Autodesk Fusion 360 part; units mm, degrees
(part 4 of 7)
  spline S11 degree 5 poles (-8.4802, -4.8873) (-8.4781, -4.8839) (-8.474, -4.8771) (-8.4679, -4.8668) (-8.4597, -4.8532) (-8.4496, -4.8361) (-8.4397, -4.8189) (-8.4298, -4.8018) (-8.42, -4.7846) (-8.4104, -4.7674) (-8.4008, -4.7502) (-8.3914, -4.733) (-8.3821, -4.7158) (-8.3729, -4.6985) (-8.3638, -4.6813) (-8.3548, -4.664) (-8.3459, -4.6467) (-8.3371, -4.6293) (-8.3285, -4.612) (-8.3199, -4.5947) (-8.3115, -4.5773) (-8.3032, -4.5599) (-8.295, -4.5426) (-8.2869, -4.5252) (-8.279, -4.5077) (-8.2711, -4.4903) (-8.2634, -4.4729) (-8.2558, -4.4554) (-8.2483, -4.438) (-8.241, -4.4205) (-8.2337, -4.403) (-8.2266, -4.3856) (-8.2196, -4.3681) (-8.2128, -4.3506) (-8.2061, -4.3331) (-8.1995, -4.3155) (-8.193, -4.298) (-8.1866, -4.2805) (-8.1804, -4.2629) (-8.1743, -4.2454) (-8.1684, -4.2279) (-8.1626, -4.2103) (-8.1569, -4.1928) (-8.1514, -4.1752) (-8.146, -4.1576) (-8.1408, -4.1401) (-8.1357, -4.1225) (-8.1307, -4.1049) (-8.1259, -4.0874) (-8.1212, -4.0698) (-8.1167, -4.0522) (-8.1124, -4.0347) (-8.1082, -4.0171) (-8.1042, -3.9995) (-8.1004, -3.982) (-8.0967, -3.9644) (-8.0932, -3.9469) (-8.0898, -3.9293) (-8.0866, -3.9118) (-8.0836, -3.8943) (-8.0808, -3.8768) (-8.0783, -3.8592) (-8.076, -3.8417) (-8.074, -3.8243) (-8.0722, -3.8068) (-8.0706, -3.7893) (-8.0691, -3.7719) (-8.0678, -3.7545) (-8.0667, -3.7371) (-8.0658, -3.7197) (-8.0656, -3.7024) (-8.066, -3.6885) (-8.0667, -3.6782) (-8.0674, -3.6713) (-8.0678, -3.6679) knots -1 -1 -1 -1 -1 -1 -0.98571429 -0.97142857 -0.95714286 -0.94285714 -0.92857143 -0.91428571 -0.9 -0.88571429 -0.87142857 -0.85714286 -0.84285714 -0.82857143 -0.81428571 -0.8 -0.78571429 -0.77142857 -0.75714286 -0.74285714 -0.72857143 -0.71428571 -0.7 -0.68571429 -0.67142857 -0.65714286 -0.64285714 -0.62857143 -0.61428571 -0.6 -0.58571429 -0.57142857 -0.55714286 -0.54285714 -0.52857143 -0.51428571 -0.5 -0.48571429 -0.47142857 -0.45714286 -0.44285714 -0.42857143 -0.41428571 -0.4 -0.38571429 -0.37142857 -0.35714286 -0.34285714 -0.32857143 -0.31428571 -0.3 -0.28571429 -0.27142857 -0.25714286 -0.24285714 -0.22857143 -0.21428571 -0.2 -0.18571429 -0.17142857 -0.15714286 -0.14285714 -0.12857143 -0.11428571 -0.1 -0.08571429 -0.07142857 -0.05714286 -0.04285714 -0.02857143 -0.01428571 0 0 0 0 0 0
  line L17 (-8.0678, -3.6679) -> (-8.1065, -3.3269)
  arc A18 (-7.9374, -3.1065) -> (-8.1065, -3.3269) centre (-7.9078, -3.3043) ccw
  line L18 (-7.9374, -3.1065) -> (-7.0422, -3.1065)
  arc A19 (-6.8731, -3.3269) -> (-7.0422, -3.1065) centre (-7.0718, -3.3043) ccw
  line L19 (-6.8731, -3.3269) -> (-6.9118, -3.6679)
  spline S12 degree 5 poles (-6.9118, -3.6679) (-6.9122, -3.6713) (-6.9128, -3.6782) (-6.9136, -3.6885) (-6.914, -3.7024) (-6.9138, -3.7197) (-6.9129, -3.7371) (-6.9118, -3.7545) (-6.9105, -3.7719) (-6.909, -3.7893) (-6.9074, -3.8068) (-6.9056, -3.8243) (-6.9036, -3.8417) (-6.9013, -3.8592) (-6.8988, -3.8768) (-6.896, -3.8943) (-6.893, -3.9118) (-6.8898, -3.9293) (-6.8864, -3.9469) (-6.8829, -3.9644) (-6.8792, -3.982) (-6.8754, -3.9995) (-6.8714, -4.0171) (-6.8672, -4.0347) (-6.8629, -4.0522) (-6.8584, -4.0698) (-6.8537, -4.0874) (-6.8489, -4.1049) (-6.8439, -4.1225) (-6.8388, -4.1401) (-6.8336, -4.1576) (-6.8282, -4.1752) (-6.8227, -4.1928) (-6.817, -4.2103) (-6.8112, -4.2279) (-6.8053, -4.2454) (-6.7992, -4.2629) (-6.793, -4.2805) (-6.7866, -4.298) (-6.7801, -4.3155) (-6.7735, -4.3331) (-6.7668, -4.3506) (-6.76, -4.3681) (-6.753, -4.3856) (-6.7459, -4.403) (-6.7386, -4.4205) (-6.7313, -4.438) (-6.7238, -4.4554) (-6.7162, -4.4729) (-6.7085, -4.4903) (-6.7006, -4.5077) (-6.6927, -4.5252) (-6.6846, -4.5426) (-6.6764, -4.5599) (-6.6681, -4.5773) (-6.6597, -4.5947) (-6.6511, -4.612) (-6.6425, -4.6293) (-6.6337, -4.6467) (-6.6248, -4.664) (-6.6158, -4.6813) (-6.6067, -4.6985) (-6.5975, -4.7158) (-6.5882, -4.733) (-6.5788, -4.7502) (-6.5692, -4.7674) (-6.5596, -4.7846) (-6.5498, -4.8018) (-6.5399, -4.8189) (-6.53, -4.8361) (-6.5199, -4.8532) (-6.5117, -4.8668) (-6.5056, -4.8771) (-6.5015, -4.8839) (-6.4994, -4.8873) knots 0 0 0 0 0 0 0.01428571 0.02857143 0.04285714 0.05714286 0.07142857 0.08571429 0.1 0.11428571 0.12857143 0.14285714 0.15714286 0.17142857 0.18571429 0.2 0.21428571 0.22857143 0.24285714 0.25714286 0.27142857 0.28571429 0.3 0.31428571 0.32857143 0.34285714 0.35714286 0.37142857 0.38571429 0.4 0.41428571 0.42857143 0.44285714 0.45714286 0.47142857 0.48571429 0.5 0.51428571 0.52857143 0.54285714 0.55714286 0.57142857 0.58571429 0.6 0.61428571 0.62857143 0.64285714 0.65714286 0.67142857 0.68571429 0.7 0.71428571 0.72857143 0.74285714 0.75714286 0.77142857 0.78571429 0.8 0.81428571 0.82857143 0.84285714 0.85714286 0.87142857 0.88571429 0.9 0.91428571 0.92857143 0.94285714 0.95714286 0.97142857 0.98571429 1 1 1 1 1 1
  arc A20 (-6.4994, -4.8873) -> (-5.9669, -4.8873) centre (-6.2332, 2.3078) ccw
  spline S13 degree 5 poles (-5.9669, -4.8873) (-5.9649, -4.8839) (-5.9607, -4.8771) (-5.9546, -4.8668) (-5.9464, -4.8532) (-5.9364, -4.8361) (-5.9264, -4.8189) (-5.9165, -4.8018) (-5.9067, -4.7846) (-5.8971, -4.7674) (-5.8876, -4.7502) (-5.8781, -4.733) (-5.8688, -4.7158) (-5.8596, -4.6985) (-5.8505, -4.6813) (-5.8415, -4.664) (-5.8326, -4.6467) (-5.8238, -4.6293) (-5.8152, -4.612) (-5.8067, -4.5947) (-5.7982, -4.5773) (-5.7899, -4.5599) (-5.7817, -4.5426) (-5.7737, -4.5252) (-5.7657, -4.5077) (-5.7579, -4.4903) (-5.7501, -4.4729) (-5.7425, -4.4554) (-5.7351, -4.438) (-5.7277, -4.4205) (-5.7205, -4.403) (-5.7134, -4.3856) (-5.7064, -4.3681) (-5.6995, -4.3506) (-5.6928, -4.3331) (-5.6862, -4.3155) (-5.6797, -4.298) (-5.6734, -4.2805) (-5.6672, -4.2629) (-5.6611, -4.2454) (-5.6551, -4.2279) (-5.6493, -4.2103) (-5.6437, -4.1928) (-5.6381, -4.1752) (-5.6327, -4.1576) (-5.6275, -4.1401) (-5.6224, -4.1225) (-5.6174, -4.1049) (-5.6126, -4.0874) (-5.608, -4.0698) (-5.6035, -4.0522) (-5.5991, -4.0347) (-5.5949, -4.0171) (-5.5909, -3.9995) (-5.5871, -3.982) (-5.5835, -3.9644) (-5.5799, -3.9469) (-5.5766, -3.9293) (-5.5734, -3.9118) (-5.5703, -3.8943) (-5.5675, -3.8768) (-5.565, -3.8592) (-5.5627, -3.8417) (-5.5607, -3.8243) (-5.5589, -3.8068) (-5.5573, -3.7893) (-5.5559, -3.7719) (-5.5545, -3.7545) (-5.5534, -3.7371) (-5.5526, -3.7197) (-5.5523, -3.7024) (-5.5527, -3.6885) (-5.5535, -3.6782) (-5.5542, -3.6713) (-5.5545, -3.6679) knots -1 -1 -1 -1 -1 -1 -0.98571429 -0.97142857 -0.95714286 -0.94285714 -0.92857143 -0.91428571 -0.9 -0.88571429 -0.87142857 -0.85714286 -0.84285714 -0.82857143 -0.81428571 -0.8 -0.78571429 -0.77142857 -0.75714286 -0.74285714 -0.72857143 -0.71428571 -0.7 -0.68571429 -0.67142857 -0.65714286 -0.64285714 -0.62857143 -0.61428571 -0.6 -0.58571429 -0.57142857 -0.55714286 -0.54285714 -0.52857143 -0.51428571 -0.5 -0.48571429 -0.47142857 -0.45714286 -0.44285714 -0.42857143 -0.41428571 -0.4 -0.38571429 -0.37142857 -0.35714286 -0.34285714 -0.32857143 -0.31428571 -0.3 -0.28571429 -0.27142857 -0.25714286 -0.24285714 -0.22857143 -0.21428571 -0.2 -0.18571429 -0.17142857 -0.15714286 -0.14285714 -0.12857143 -0.11428571 -0.1 -0.08571429 -0.07142857 -0.05714286 -0.04285714 -0.02857143 -0.01428571 0 0 0 0 0 0
  line L20 (-5.5545, -3.6679) -> (-5.5933, -3.3269)
  arc A21 (-5.4241, -3.1065) -> (-5.5933, -3.3269) centre (-5.3945, -3.3043) ccw
  line L21 (-5.4241, -3.1065) -> (-4.5289, -3.1065)
  arc A22 (-4.3598, -3.3269) -> (-4.5289, -3.1065) centre (-4.5585, -3.3043) ccw
  line L22 (-4.3598, -3.3269) -> (-4.3985, -3.6679)
  spline S14 degree 5 poles (-4.3985, -3.6679) (-4.3989, -3.6713) (-4.3996, -3.6782) (-4.4003, -3.6885) (-4.4007, -3.7024) (-4.4005, -3.7197) (-4.3997, -3.7371) (-4.3985, -3.7545) (-4.3972, -3.7719) (-4.3957, -3.7893) (-4.3941, -3.8068) (-4.3923, -3.8243) (-4.3903, -3.8417) (-4.3881, -3.8592) (-4.3855, -3.8768) (-4.3827, -3.8943) (-4.3797, -3.9118) (-4.3765, -3.9293) (-4.3731, -3.9469) (-4.3696, -3.9644) (-4.3659, -3.982) (-4.3621, -3.9995) (-4.3581, -4.0171) (-4.3539, -4.0347) (-4.3496, -4.0522) (-4.3451, -4.0698) (-4.3404, -4.0874) (-4.3356, -4.1049) (-4.3307, -4.1225) (-4.3255, -4.1401) (-4.3203, -4.1576) (-4.3149, -4.1752) (-4.3094, -4.1928) (-4.3037, -4.2103) (-4.2979, -4.2279) (-4.292, -4.2454) (-4.2859, -4.2629) (-4.2797, -4.2805) (-4.2733, -4.298) (-4.2669, -4.3155) (-4.2603, -4.3331) (-4.2535, -4.3506) (-4.2467, -4.3681) (-4.2397, -4.3856) (-4.2326, -4.403) (-4.2253, -4.4205) (-4.218, -4.438) (-4.2105, -4.4554) (-4.2029, -4.4729) (-4.1952, -4.4903) (-4.1874, -4.5077) (-4.1794, -4.5252) (-4.1713, -4.5426) (-4.1631, -4.5599) (-4.1548, -4.5773) (-4.1464, -4.5947) (-4.1379, -4.612) (-4.1292, -4.6293) (-4.1204, -4.6467) (-4.1116, -4.664) (-4.1026, -4.6813) (-4.0935, -4.6985) (-4.0843, -4.7158) (-4.0749, -4.733) (-4.0655, -4.7502) (-4.056, -4.7674) (-4.0463, -4.7846) (-4.0365, -4.8018) (-4.0267, -4.8189) (-4.0167, -4.8361) (-4.0066, -4.8532) (-3.9985, -4.8668) (-3.9923, -4.8771) (-3.9882, -4.8839) (-3.9861, -4.8873) knots 0 0 0 0 0 0 0.01428571 0.02857143 0.04285714 0.05714286 0.07142857 0.08571429 0.1 0.11428571 0.12857143 0.14285714 0.15714286 0.17142857 0.18571429 0.2 0.21428571 0.22857143 0.24285714 0.25714286 0.27142857 0.28571429 0.3 0.31428571 0.32857143 0.34285714 0.35714286 0.37142857 0.38571429 0.4 0.41428571 0.42857143 0.44285714 0.45714286 0.47142857 0.48571429 0.5 0.51428571 0.52857143 0.54285714 0.55714286 0.57142857 0.58571429 0.6 0.61428571 0.62857143 0.64285714 0.65714286 0.67142857 0.68571429 0.7 0.71428571 0.72857143 0.74285714 0.75714286 0.77142857 0.78571429 0.8 0.81428571 0.82857143 0.84285714 0.85714286 0.87142857 0.88571429 0.9 0.91428571 0.92857143 0.94285714 0.95714286 0.97142857 0.98571429 1 1 1 1 1 1
  arc A23 (-3.9861, -4.8873) -> (-3.4537, -4.8873) centre (-3.7199, 2.3078) ccw
  spline S15 degree 5 poles (-3.4537, -4.8873) (-3.4516, -4.8839) (-3.4475, -4.8771) (-3.4413, -4.8668) (-3.4332, -4.8532) (-3.4231, -4.8361) (-3.4131, -4.8189) (-3.4032, -4.8018) (-3.3935, -4.7846) (-3.3838, -4.7674) (-3.3743, -4.7502) (-3.3648, -4.733) (-3.3555, -4.7158) (-3.3463, -4.6985) (-3.3372, -4.6813) (-3.3282, -4.664) (-3.3193, -4.6467) (-3.3106, -4.6293) (-3.3019, -4.612) (-3.2934, -4.5947) (-3.285, -4.5773) (-3.2766, -4.5599) (-3.2685, -4.5426) (-3.2604, -4.5252) (-3.2524, -4.5077) (-3.2446, -4.4903) (-3.2369, -4.4729) (-3.2293, -4.4554) (-3.2218, -4.438) (-3.2144, -4.4205) (-3.2072, -4.403) (-3.2001, -4.3856) (-3.1931, -4.3681) (-3.1862, -4.3506) (-3.1795, -4.3331) (-3.1729, -4.3155) (-3.1664, -4.298) (-3.1601, -4.2805) (-3.1539, -4.2629) (-3.1478, -4.2454) (-3.1419, -4.2279) (-3.136, -4.2103) (-3.1304, -4.1928) (-3.1249, -4.1752) (-3.1195, -4.1576) (-3.1142, -4.1401) (-3.1091, -4.1225) (-3.1042, -4.1049) (-3.0993, -4.0874) (-3.0947, -4.0698) (-3.0902, -4.0522) (-3.0858, -4.0347) (-3.0817, -4.0171) (-3.0777, -3.9995) (-3.0738, -3.982) (-3.0702, -3.9644) (-3.0667, -3.9469) (-3.0633, -3.9293) (-3.0601, -3.9118) (-3.0571, -3.8943) (-3.0543, -3.8768) (-3.0517, -3.8592) (-3.0495, -3.8417) (-3.0474, -3.8243) (-3.0457, -3.8068) (-3.0441, -3.7893) (-3.0426, -3.7719) (-3.0413, -3.7545) (-3.0401, -3.7371) (-3.0393, -3.7197) (-3.0391, -3.7024) (-3.0395, -3.6885) (-3.0402, -3.6782) (-3.0409, -3.6713) (-3.0413, -3.6679) knots -1 -1 -1 -1 -1 -1 -0.98571429 -0.97142857 -0.95714286 -0.94285714 -0.92857143 -0.91428571 -0.9 -0.88571429 -0.87142857 -0.85714286 -0.84285714 -0.82857143 -0.81428571 -0.8 -0.78571429 -0.77142857 -0.75714286 -0.74285714 -0.72857143 -0.71428571 -0.7 -0.68571429 -0.67142857 -0.65714286 -0.64285714 -0.62857143 -0.61428571 -0.6 -0.58571429 -0.57142857 -0.55714286 -0.54285714 -0.52857143 -0.51428571 -0.5 -0.48571429 -0.47142857 -0.45714286 -0.44285714 -0.42857143 -0.41428571 -0.4 -0.38571429 -0.37142857 -0.35714286 -0.34285714 -0.32857143 -0.31428571 -0.3 -0.28571429 -0.27142857 -0.25714286 -0.24285714 -0.22857143 -0.21428571 -0.2 -0.18571429 -0.17142857 -0.15714286 -0.14285714 -0.12857143 -0.11428571 -0.1 -0.08571429 -0.07142857 -0.05714286 -0.04285714 -0.02857143 -0.01428571 0 0 0 0 0 0
  line L23 (-3.0413, -3.6679) -> (-3.08, -3.3269)
  arc A24 (-2.9108, -3.1065) -> (-3.08, -3.3269) centre (-2.8813, -3.3043) ccw
  line L24 (-2.9108, -3.1065) -> (-2.0157, -3.1065)
  arc A25 (-1.8465, -3.3269) -> (-2.0157, -3.1065) centre (-2.0452, -3.3043) ccw
  line L25 (-1.8465, -3.3269) -> (-1.8852, -3.6679)
  spline S16 degree 5 poles (-1.8852, -3.6679) (-1.8856, -3.6713) (-1.8863, -3.6782) (-1.887, -3.6885) (-1.8874, -3.7024) (-1.8872, -3.7197) (-1.8864, -3.7371) (-1.8852, -3.7545) (-1.8839, -3.7719) (-1.8824, -3.7893) (-1.8808, -3.8068) (-1.8791, -3.8243) (-1.877, -3.8417) (-1.8748, -3.8592) (-1.8722, -3.8768) (-1.8694, -3.8943) (-1.8664, -3.9118) (-1.8632, -3.9293) (-1.8598, -3.9469) (-1.8563, -3.9644) (-1.8527, -3.982) (-1.8488, -3.9995) (-1.8448, -4.0171) (-1.8407, -4.0347) (-1.8363, -4.0522) (-1.8318, -4.0698) (-1.8272, -4.0874) (-1.8223, -4.1049) (-1.8174, -4.1225) (-1.8123, -4.1401) (-1.807, -4.1576) (-1.8016, -4.1752) (-1.7961, -4.1928) (-1.7905, -4.2103) (-1.7846, -4.2279) (-1.7787, -4.2454) (-1.7726, -4.2629) (-1.7664, -4.2805) (-1.7601, -4.298) (-1.7536, -4.3155) (-1.747, -4.3331) (-1.7403, -4.3506) (-1.7334, -4.3681) (-1.7264, -4.3856) (-1.7193, -4.403) (-1.7121, -4.4205) (-1.7047, -4.438) (-1.6972, -4.4554) (-1.6896, -4.4729) (-1.6819, -4.4903) (-1.6741, -4.5077) (-1.6661, -4.5252) (-1.6581, -4.5426) (-1.6499, -4.5599) (-1.6415, -4.5773) (-1.6331, -4.5947) (-1.6246, -4.612) (-1.6159, -4.6293) (-1.6072, -4.6467) (-1.5983, -4.664) (-1.5893, -4.6813) (-1.5802, -4.6985) (-1.571, -4.7158) (-1.5617, -4.733) (-1.5522, -4.7502) (-1.5427, -4.7674) (-1.533, -4.7846) (-1.5233, -4.8018) (-1.5134, -4.8189) (-1.5034, -4.8361) (-1.4933, -4.8532) (-1.4852, -4.8668) (-1.479, -4.8771) (-1.4749, -4.8839) (-1.4728, -4.8873) knots 0 0 0 0 0 0 0.01428571 0.02857143 0.04285714 0.05714286 0.07142857 0.08571429 0.1 0.11428571 0.12857143 0.14285714 0.15714286 0.17142857 0.18571429 0.2 0.21428571 0.22857143 0.24285714 0.25714286 0.27142857 0.28571429 0.3 0.31428571 0.32857143 0.34285714 0.35714286 0.37142857 0.38571429 0.4 0.41428571 0.42857143 0.44285714 0.45714286 0.47142857 0.48571429 0.5 0.51428571 0.52857143 0.54285714 0.55714286 0.57142857 0.58571429 0.6 0.61428571 0.62857143 0.64285714 0.65714286 0.67142857 0.68571429 0.7 0.71428571 0.72857143 0.74285714 0.75714286 0.77142857 0.78571429 0.8 0.81428571 0.82857143 0.84285714 0.85714286 0.87142857 0.88571429 0.9 0.91428571 0.92857143 0.94285714 0.95714286 0.97142857 0.98571429 1 1 1 1 1 1
  arc A26 (-1.4728, -4.8873) -> (-0.9404, -4.8873) centre (-1.2066, 2.3078) ccw
  spline S17 degree 5 poles (-0.9404, -4.8873) (-0.9383, -4.8839) (-0.9342, -4.8771) (-0.928, -4.8668) (-0.9199, -4.8532) (-0.9098, -4.8361) (-0.8998, -4.8189) (-0.89, -4.8018) (-0.8802, -4.7846) (-0.8705, -4.7674) (-0.861, -4.7502) (-0.8516, -4.733) (-0.8422, -4.7158) (-0.833, -4.6985) (-0.8239, -4.6813) (-0.8149, -4.664) (-0.8061, -4.6467) (-0.7973, -4.6293) (-0.7886, -4.612) (-0.7801, -4.5947) (-0.7717, -4.5773) (-0.7634, -4.5599) (-0.7552, -4.5426) (-0.7471, -4.5252) (-0.7391, -4.5077) (-0.7313, -4.4903) (-0.7236, -4.4729) (-0.716, -4.4554) (-0.7085, -4.438) (-0.7012, -4.4205) (-0.6939, -4.403) (-0.6868, -4.3856) (-0.6798, -4.3681) (-0.673, -4.3506) (-0.6662, -4.3331) (-0.6596, -4.3155) (-0.6532, -4.298) (-0.6468, -4.2805) (-0.6406, -4.2629) (-0.6345, -4.2454) (-0.6286, -4.2279) (-0.6228, -4.2103) (-0.6171, -4.1928) (-0.6116, -4.1752) (-0.6062, -4.1576) (-0.601, -4.1401) (-0.5958, -4.1225) (-0.5909, -4.1049) (-0.5861, -4.0874) (-0.5814, -4.0698) (-0.5769, -4.0522) (-0.5726, -4.0347) (-0.5684, -4.0171) (-0.5644, -3.9995) (-0.5606, -3.982) (-0.5569, -3.9644) (-0.5534, -3.9469) (-0.55, -3.9293) (-0.5468, -3.9118) (-0.5438, -3.8943) (-0.541, -3.8768) (-0.5384, -3.8592) (-0.5362, -3.8417) (-0.5342, -3.8243) (-0.5324, -3.8068) (-0.5308, -3.7893) (-0.5293, -3.7719) (-0.528, -3.7545) (-0.5268, -3.7371) (-0.526, -3.7197) (-0.5258, -3.7024) (-0.5262, -3.6885) (-0.5269, -3.6782) (-0.5276, -3.6713) (-0.528, -3.6679) knots -1 -1 -1 -1 -1 -1 -0.98571429 -0.97142857 -0.95714286 -0.94285714 -0.92857143 -0.91428571 -0.9 -0.88571429 -0.87142857 -0.85714286 -0.84285714 -0.82857143 -0.81428571 -0.8 -0.78571429 -0.77142857 -0.75714286 -0.74285714 -0.72857143 -0.71428571 -0.7 -0.68571429 -0.67142857 -0.65714286 -0.64285714 -0.62857143 -0.61428571 -0.6 -0.58571429 -0.57142857 -0.55714286 -0.54285714 -0.52857143 -0.51428571 -0.5 -0.48571429 -0.47142857 -0.45714286 -0.44285714 -0.42857143 -0.41428571 -0.4 -0.38571429 -0.37142857 -0.35714286 -0.34285714 -0.32857143 -0.31428571 -0.3 -0.28571429 -0.27142857 -0.25714286 -0.24285714 -0.22857143 -0.21428571 -0.2 -0.18571429 -0.17142857 -0.15714286 -0.14285714 -0.12857143 -0.11428571 -0.1 -0.08571429 -0.07142857 -0.05714286 -0.04285714 -0.02857143 -0.01428571 0 0 0 0 0 0
  line L26 (-0.528, -3.6679) -> (-0.5667, -3.3269)
  arc A27 (-0.3976, -3.1065) -> (-0.5667, -3.3269) centre (-0.368, -3.3043) ccw
  line L27 (-0.3976, -3.1065) -> (0.4976, -3.1065)
  arc A28 (0.6668, -3.3269) -> (0.4976, -3.1065) centre (0.468, -3.3043) ccw
  line L28 (0.6668, -3.3269) -> (0.628, -3.6679)
  spline S18 degree 5 poles (0.628, -3.6679) (0.6277, -3.6713) (0.627, -3.6782) (0.6262, -3.6885) (0.6258, -3.7024) (0.6261, -3.7197) (0.6269, -3.7371) (0.628, -3.7545) (0.6294, -3.7719) (0.6308, -3.7893) (0.6324, -3.8068) (0.6342, -3.8243) (0.6362, -3.8417) (0.6385, -3.8592) (0.641, -3.8768) (0.6438, -3.8943) (0.6469, -3.9118) (0.6501, -3.9293) (0.6534, -3.9469) (0.657, -3.9644) (0.6606, -3.982) (0.6644, -3.9995) (0.6684, -4.0171) (0.6726, -4.0347) (0.677, -4.0522) (0.6815, -4.0698) (0.6861, -4.0874) (0.6909, -4.1049) (0.6959, -4.1225) (0.701, -4.1401) (0.7062, -4.1576) (0.7116, -4.1752) (0.7172, -4.1928) (0.7228, -4.2103) (0.7286, -4.2279) (0.7346, -4.2454) (0.7406, -4.2629) (0.7469, -4.2805) (0.7532, -4.298) (0.7597, -4.3155) (0.7663, -4.3331) (0.773, -4.3506) (0.7799, -4.3681) (0.7869, -4.3856) (0.794, -4.403) (0.8012, -4.4205) (0.8086, -4.438) (0.816, -4.4554) (0.8236, -4.4729) (0.8314, -4.4903) (0.8392, -4.5077) (0.8471, -4.5252) (0.8552, -4.5426) (0.8634, -4.5599) (0.8717, -4.5773) (0.8801, -4.5947) (0.8887, -4.612) (0.8973, -4.6293) (0.9061, -4.6467) (0.915, -4.664) (0.924, -4.6813) (0.9331, -4.6985) (0.9423, -4.7158) (0.9516, -4.733) (0.9611, -4.7502) (0.9706, -4.7674) (0.9802, -4.7846) (0.99, -4.8018) (0.9999, -4.8189) (1.0099, -4.8361) (1.0199, -4.8532) (1.0281, -4.8668) (1.0342, -4.8771) (1.0384, -4.8839) (1.0404, -4.8873) knots 0 0 0 0 0 0 0.01428571 0.02857143 0.04285714 0.05714286 0.07142857 0.08571429 0.1 0.11428571 0.12857143 0.14285714 0.15714286 0.17142857 0.18571429 0.2 0.21428571 0.22857143 0.24285714 0.25714286 0.27142857 0.28571429 0.3 0.31428571 0.32857143 0.34285714 0.35714286 0.37142857 0.38571429 0.4 0.41428571 0.42857143 0.44285714 0.45714286 0.47142857 0.48571429 0.5 0.51428571 0.52857143 0.54285714 0.55714286 0.57142857 0.58571429 0.6 0.61428571 0.62857143 0.64285714 0.65714286 0.67142857 0.68571429 0.7 0.71428571 0.72857143 0.74285714 0.75714286 0.77142857 0.78571429 0.8 0.81428571 0.82857143 0.84285714 0.85714286 0.87142857 0.88571429 0.9 0.91428571 0.92857143 0.94285714 0.95714286 0.97142857 0.98571429 1 1 1 1 1 1
  arc A29 (1.0404, -4.8873) -> (1.5729, -4.8873) centre (1.3067, 2.3078) ccw
  spline S19 degree 5 poles (1.5729, -4.8873) (1.5749, -4.8839) (1.5791, -4.8771) (1.5852, -4.8668) (1.5934, -4.8532) (1.6035, -4.8361) (1.6134, -4.8189) (1.6233, -4.8018) (1.6331, -4.7846) (1.6427, -4.7674) (1.6523, -4.7502) (1.6617, -4.733) (1.671, -4.7158) (1.6802, -4.6985) (1.6893, -4.6813) (1.6983, -4.664) (1.7072, -4.6467) (1.716, -4.6293) (1.7246, -4.612) (1.7332, -4.5947) (1.7416, -4.5773) (1.7499, -4.5599) (1.7581, -4.5426) (1.7662, -4.5252) (1.7741, -4.5077) (1.782, -4.4903) (1.7897, -4.4729) (1.7973, -4.4554) (1.8048, -4.438) (1.8121, -4.4205) (1.8194, -4.403) (1.8265, -4.3856) (1.8334, -4.3681) (1.8403, -4.3506) (1.847, -4.3331) (1.8536, -4.3155) (1.8601, -4.298) (1.8665, -4.2805) (1.8727, -4.2629) (1.8788, -4.2454) (1.8847, -4.2279) (1.8905, -4.2103) (1.8962, -4.1928) (1.9017, -4.1752) (1.9071, -4.1576) (1.9123, -4.1401) (1.9174, -4.1225) (1.9224, -4.1049) (1.9272, -4.0874) (1.9319, -4.0698) (1.9364, -4.0522) (1.9407, -4.0347) (1.9449, -4.0171) (1.9489, -3.9995) (1.9527, -3.982) (1.9564, -3.9644) (1.9599, -3.9469) (1.9633, -3.9293) (1.9665, -3.9118) (1.9695, -3.8943) (1.9723, -3.8768) (1.9748, -3.8592) (1.9771, -3.8417) (1.9791, -3.8243) (1.9809, -3.8068) (1.9825, -3.7893) (1.9839, -3.7719) (1.9853, -3.7545) (1.9864, -3.7371) (1.9872, -3.7197) (1.9875, -3.7024) (1.9871, -3.6885) (1.9863, -3.6782) (1.9857, -3.6713) (1.9853, -3.6679) knots -1 -1 -1 -1 -1 -1 -0.98571429 -0.97142857 -0.95714286 -0.94285714 -0.92857143 -0.91428571 -0.9 -0.88571429 -0.87142857 -0.85714286 -0.84285714 -0.82857143 -0.81428571 -0.8 -0.78571429 -0.77142857 -0.75714286 -0.74285714 -0.72857143 -0.71428571 -0.7 -0.68571429 -0.67142857 -0.65714286 -0.64285714 -0.62857143 -0.61428571 -0.6 -0.58571429 -0.57142857 -0.55714286 -0.54285714 -0.52857143 -0.51428571 -0.5 -0.48571429 -0.47142857 -0.45714286 -0.44285714 -0.42857143 -0.41428571 -0.4 -0.38571429 -0.37142857 -0.35714286 -0.34285714 -0.32857143 -0.31428571 -0.3 -0.28571429 -0.27142857 -0.25714286 -0.24285714 -0.22857143 -0.21428571 -0.2 -0.18571429 -0.17142857 -0.15714286 -0.14285714 -0.12857143 -0.11428571 -0.1 -0.08571429 -0.07142857 -0.05714286 -0.04285714 -0.02857143 -0.01428571 0 0 0 0 0 0
  line L29 (1.9853, -3.6679) -> (1.9466, -3.3269)
  arc A30 (2.1157, -3.1065) -> (1.9466, -3.3269) centre (2.1453, -3.3043) ccw
  line L30 (2.1157, -3.1065) -> (3.0109, -3.1065)
  arc A31 (3.18, -3.3269) -> (3.0109, -3.1065) centre (2.9813, -3.3043) ccw
  line L31 (3.18, -3.3269) -> (3.1413, -3.6679)
  spline S20 degree 5 poles (3.1413, -3.6679) (3.1409, -3.6713) (3.1402, -3.6782) (3.1395, -3.6885) (3.1391, -3.7024) (3.1393, -3.7197) (3.1402, -3.7371) (3.1413, -3.7545) (3.1426, -3.7719) (3.1441, -3.7893) (3.1457, -3.8068) (3.1475, -3.8243) (3.1495, -3.8417) (3.1518, -3.8592) (3.1543, -3.8768) (3.1571, -3.8943) (3.1601, -3.9118) (3.1633, -3.9293) (3.1667, -3.9469) (3.1702, -3.9644) (3.1739, -3.982) (3.1777, -3.9995) (3.1817, -4.0171) (3.1859, -4.0347) (3.1902, -4.0522) (3.1947, -4.0698) (3.1994, -4.0874) (3.2042, -4.1049) (3.2092, -4.1225) (3.2143, -4.1401) (3.2195, -4.1576) (3.2249, -4.1752) (3.2304, -4.1928) (3.2361, -4.2103) (3.2419, -4.2279) (3.2478, -4.2454) (3.2539, -4.2629) (3.2601, -4.2805) (3.2665, -4.298) (3.273, -4.3155) (3.2796, -4.3331) (3.2863, -4.3506) (3.2931, -4.3681) (3.3001, -4.3856) (3.3072, -4.403) (3.3145, -4.4205) (3.3218, -4.438) (3.3293, -4.4554) (3.3369, -4.4729) (3.3446, -4.4903) (3.3525, -4.5077) (3.3604, -4.5252) (3.3685, -4.5426) (3.3767, -4.5599) (3.385, -4.5773) (3.3934, -4.5947) (3.402, -4.612) (3.4106, -4.6293) (3.4194, -4.6467) (3.4283, -4.664) (3.4373, -4.6813) (3.4464, -4.6985) (3.4556, -4.7158) (3.4649, -4.733) (3.4743, -4.7502) (3.4839, -4.7674) (3.4935, -4.7846) (3.5033, -4.8018) (3.5131, -4.8189) (3.5231, -4.8361) (3.5332, -4.8532) (3.5414, -4.8668) (3.5475, -4.8771) (3.5516, -4.8839) (3.5537, -4.8873) knots 0 0 0 0 0 0 0.01428571 0.02857143 0.04285714 0.05714286 0.07142857 0.08571429 0.1 0.11428571 0.12857143 0.14285714 0.15714286 0.17142857 0.18571429 0.2 0.21428571 0.22857143 0.24285714 0.25714286 0.27142857 0.28571429 0.3 0.31428571 0.32857143 0.34285714 0.35714286 0.37142857 0.38571429 0.4 0.41428571 0.42857143 0.44285714 0.45714286 0.47142857 0.48571429 0.5 0.51428571 0.52857143 0.54285714 0.55714286 0.57142857 0.58571429 0.6 0.61428571 0.62857143 0.64285714 0.65714286 0.67142857 0.68571429 0.7 0.71428571 0.72857143 0.74285714 0.75714286 0.77142857 0.78571429 0.8 0.81428571 0.82857143 0.84285714 0.85714286 0.87142857 0.88571429 0.9 0.91428571 0.92857143 0.94285714 0.95714286 0.97142857 0.98571429 1 1 1 1 1 1
  arc A32 (3.5537, -4.8873) -> (4.0862, -4.8873) centre (3.8199, 2.3078) ccw
  spline S21 degree 5 poles (4.0862, -4.8873) (4.0882, -4.8839) (4.0924, -4.8771) (4.0985, -4.8668) (4.1067, -4.8532) (4.1167, -4.8361) (4.1267, -4.8189) (4.1366, -4.8018) (4.1463, -4.7846) (4.156, -4.7674) (4.1655, -4.7502) (4.175, -4.733) (4.1843, -4.7158) (4.1935, -4.6985) (4.2026, -4.6813) (4.2116, -4.664) (4.2205, -4.6467) (4.2293, -4.6293) (4.2379, -4.612) (4.2464, -4.5947) (4.2549, -4.5773) (4.2632, -4.5599) (4.2714, -4.5426) (4.2794, -4.5252) (4.2874, -4.5077) (4.2952, -4.4903) (4.303, -4.4729) (4.3106, -4.4554) (4.318, -4.438) (4.3254, -4.4205) (4.3326, -4.403) (4.3397, -4.3856) (4.3467, -4.3681) (4.3536, -4.3506) (4.3603, -4.3331) (4.3669, -4.3155) (4.3734, -4.298) (4.3797, -4.2805) (4.3859, -4.2629) (4.392, -4.2454) (4.398, -4.2279) (4.4038, -4.2103) (4.4094, -4.1928) (4.415, -4.1752) (4.4204, -4.1576) (4.4256, -4.1401) (4.4307, -4.1225) (4.4357, -4.1049) (4.4405, -4.0874) (4.4451, -4.0698) (4.4496, -4.0522) (4.454, -4.0347) (4.4582, -4.0171) (4.4621, -3.9995) (4.466, -3.982) (4.4696, -3.9644) (4.4732, -3.9469) (4.4765, -3.9293) (4.4797, -3.9118) (4.4828, -3.8943) (4.4856, -3.8768) (4.4881, -3.8592) (4.4904, -3.8417) (4.4924, -3.8243) (4.4941, -3.8068) (4.4958, -3.7893) (4.4972, -3.7719) (4.4986, -3.7545) (4.4997, -3.7371) (4.5005, -3.7197) (4.5008, -3.7024) (4.5004, -3.6885) (4.4996, -3.6782) (4.4989, -3.6713) (4.4985, -3.6679) knots -1 -1 -1 -1 -1 -1 -0.98571429 -0.97142857 -0.95714286 -0.94285714 -0.92857143 -0.91428571 -0.9 -0.88571429 -0.87142857 -0.85714286 -0.84285714 -0.82857143 -0.81428571 -0.8 -0.78571429 -0.77142857 -0.75714286 -0.74285714 -0.72857143 -0.71428571 -0.7 -0.68571429 -0.67142857 -0.65714286 -0.64285714 -0.62857143 -0.61428571 -0.6 -0.58571429 -0.57142857 -0.55714286 -0.54285714 -0.52857143 -0.51428571 -0.5 -0.48571429 -0.47142857 -0.45714286 -0.44285714 -0.42857143 -0.41428571 -0.4 -0.38571429 -0.37142857 -0.35714286 -0.34285714 -0.32857143 -0.31428571 -0.3 -0.28571429 -0.27142857 -0.25714286 -0.24285714 -0.22857143 -0.21428571 -0.2 -0.18571429 -0.17142857 -0.15714286 -0.14285714 -0.12857143 -0.11428571 -0.1 -0.08571429 -0.07142857 -0.05714286 -0.04285714 -0.02857143 -0.01428571 0 0 0 0 0 0
  line L32 (4.4985, -3.6679) -> (4.4598, -3.3269)
  arc A33 (4.629, -3.1065) -> (4.4598, -3.3269) centre (4.6585, -3.3043) ccw
  line L33 (4.629, -3.1065) -> (5.5242, -3.1065)
  arc A34 (5.6933, -3.3269) -> (5.5242, -3.1065) centre (5.4946, -3.3043) ccw
  line L34 (5.6933, -3.3269) -> (5.6546, -3.6679)
  spline S22 degree 5 poles (5.6546, -3.6679) (5.6542, -3.6713) (5.6535, -3.6782) (5.6528, -3.6885) (5.6524, -3.7024) (5.6526, -3.7197) (5.6534, -3.7371) (5.6546, -3.7545) (5.6559, -3.7719) (5.6574, -3.7893) (5.659, -3.8068) (5.6608, -3.8243) (5.6628, -3.8417) (5.665, -3.8592) (5.6676, -3.8768) (5.6704, -3.8943) (5.6734, -3.9118) (5.6766, -3.9293) (5.68, -3.9469) (5.6835, -3.9644) (5.6872, -3.982) (5.691, -3.9995) (5.695, -4.0171) (5.6992, -4.0347) (5.7035, -4.0522) (5.708, -4.0698) (5.7127, -4.0874) (5.7175, -4.1049) (5.7224, -4.1225) (5.7275, -4.1401) (5.7328, -4.1576) (5.7382, -4.1752) (5.7437, -4.1928) (5.7494, -4.2103) (5.7552, -4.2279) (5.7611, -4.2454) (5.7672, -4.2629) (5.7734, -4.2805) (5.7798, -4.298) (5.7862, -4.3155) (5.7928, -4.3331) (5.7996, -4.3506) (5.8064, -4.3681) (5.8134, -4.3856) (5.8205, -4.403) (5.8277, -4.4205) (5.8351, -4.438) (5.8426, -4.4554) (5.8502, -4.4729) (5.8579, -4.4903) (5.8657, -4.5077) (5.8737, -4.5252) (5.8818, -4.5426) (5.89, -4.5599) (5.8983, -4.5773) (5.9067, -4.5947) (5.9152, -4.612) (5.9239, -4.6293) (5.9327, -4.6467) (5.9415, -4.664) (5.9505, -4.6813) (5.9596, -4.6985) (5.9688, -4.7158) (5.9782, -4.733) (5.9876, -4.7502) (5.9971, -4.7674) (6.0068, -4.7846) (6.0166, -4.8018) (6.0264, -4.8189) (6.0364, -4.8361) (6.0465, -4.8532) (6.0546, -4.8668) (6.0608, -4.8771) (6.0649, -4.8839) (6.067, -4.8873) knots 0 0 0 0 0 0 0.01428571 0.02857143 0.04285714 0.05714286 0.07142857 0.08571429 0.1 0.11428571 0.12857143 0.14285714 0.15714286 0.17142857 0.18571429 0.2 0.21428571 0.22857143 0.24285714 0.25714286 0.27142857 0.28571429 0.3 0.31428571 0.32857143 0.34285714 0.35714286 0.37142857 0.38571429 0.4 0.41428571 0.42857143 0.44285714 0.45714286 0.47142857 0.48571429 0.5 0.51428571 0.52857143 0.54285714 0.55714286 0.57142857 0.58571429 0.6 0.61428571 0.62857143 0.64285714 0.65714286 0.67142857 0.68571429 0.7 0.71428571 0.72857143 0.74285714 0.75714286 0.77142857 0.78571429 0.8 0.81428571 0.82857143 0.84285714 0.85714286 0.87142857 0.88571429 0.9 0.91428571 0.92857143 0.94285714 0.95714286 0.97142857 0.98571429 1 1 1 1 1 1
  arc A35 (6.067, -4.8873) -> (6.5994, -4.8873) centre (6.3332, 2.3078) ccw
  spline S23 degree 5 poles (6.5994, -4.8873) (6.6015, -4.8839) (6.6056, -4.8771) (6.6118, -4.8668) (6.6199, -4.8532) (6.63, -4.8361) (6.64, -4.8189) (6.6499, -4.8018) (6.6596, -4.7846) (6.6693, -4.7674) (6.6788, -4.7502) (6.6883, -4.733) (6.6976, -4.7158) (6.7068, -4.6985) (6.7159, -4.6813) (6.7249, -4.664) (6.7338, -4.6467) (6.7425, -4.6293) (6.7512, -4.612) (6.7597, -4.5947) (6.7681, -4.5773) (6.7765, -4.5599) (6.7846, -4.5426) (6.7927, -4.5252) (6.8007, -4.5077) (6.8085, -4.4903) (6.8162, -4.4729) (6.8238, -4.4554) (6.8313, -4.438) (6.8387, -4.4205) (6.8459, -4.403) (6.853, -4.3856) (6.86, -4.3681) (6.8669, -4.3506) (6.8736, -4.3331) (6.8802, -4.3155) (6.8867, -4.298) (6.893, -4.2805) (6.8992, -4.2629) (6.9053, -4.2454) (6.9112, -4.2279) (6.9171, -4.2103) (6.9227, -4.1928) (6.9282, -4.1752) (6.9336, -4.1576) (6.9389, -4.1401) (6.944, -4.1225) (6.9489, -4.1049) (6.9537, -4.0874) (6.9584, -4.0698) (6.9629, -4.0522) (6.9673, -4.0347) (6.9714, -4.0171) (6.9754, -3.9995) (6.9792, -3.982) (6.9829, -3.9644) (6.9864, -3.9469) (6.9898, -3.9293) (6.993, -3.9118) (6.996, -3.8943) (6.9988, -3.8768) (7.0014, -3.8592) (7.0036, -3.8417) (7.0056, -3.8243) (7.0074, -3.8068) (7.009, -3.7893) (7.0105, -3.7719) (7.0118, -3.7545) (7.013, -3.7371) (7.0138, -3.7197) (7.014, -3.7024) (7.0136, -3.6885) (7.0129, -3.6782) (7.0122, -3.6713) (7.0118, -3.6679) knots -1 -1 -1 -1 -1 -1 -0.98571429 -0.97142857 -0.95714286 -0.94285714 -0.92857143 -0.91428571 -0.9 -0.88571429 -0.87142857 -0.85714286 -0.84285714 -0.82857143 -0.81428571 -0.8 -0.78571429 -0.77142857 -0.75714286 -0.74285714 -0.72857143 -0.71428571 -0.7 -0.68571429 -0.67142857 -0.65714286 -0.64285714 -0.62857143 -0.61428571 -0.6 -0.58571429 -0.57142857 -0.55714286 -0.54285714 -0.52857143 -0.51428571 -0.5 -0.48571429 -0.47142857 -0.45714286 -0.44285714 -0.42857143 -0.41428571 -0.4 -0.38571429 -0.37142857 -0.35714286 -0.34285714 -0.32857143 -0.31428571 -0.3 -0.28571429 -0.27142857 -0.25714286 -0.24285714 -0.22857143 -0.21428571 -0.2 -0.18571429 -0.17142857 -0.15714286 -0.14285714 -0.12857143 -0.11428571 -0.1 -0.08571429 -0.07142857 -0.05714286 -0.04285714 -0.02857143 -0.01428571 0 0 0 0 0 0
  line L35 (7.0118, -3.6679) -> (6.9731, -3.3269)
  arc A36 (7.1423, -3.1065) -> (6.9731, -3.3269) centre (7.1718, -3.3043) ccw
  line L36 (7.1423, -3.1065) -> (8.0374, -3.1065)
  arc A37 (8.2066, -3.3269) -> (8.0374, -3.1065) centre (8.0079, -3.3043) ccw
  line L37 (8.2066, -3.3269) -> (8.1679, -3.6679)
  spline S24 degree 5 poles (8.1679, -3.6679) (8.1675, -3.6713) (8.1668, -3.6782) (8.1661, -3.6885) (8.1656, -3.7024) (8.1659, -3.7197) (8.1667, -3.7371) (8.1679, -3.7545) (8.1692, -3.7719) (8.1707, -3.7893) (8.1723, -3.8068) (8.174, -3.8243) (8.176, -3.8417) (8.1783, -3.8592) (8.1809, -3.8768) (8.1837, -3.8943) (8.1867, -3.9118) (8.1899, -3.9293) (8.1933, -3.9469) (8.1968, -3.9644) (8.2004, -3.982) (8.2043, -3.9995) (8.2083, -4.0171) (8.2124, -4.0347) (8.2168, -4.0522) (8.2213, -4.0698) (8.2259, -4.0874) (8.2308, -4.1049) (8.2357, -4.1225) (8.2408, -4.1401) (8.2461, -4.1576) (8.2514, -4.1752) (8.257, -4.1928) (8.2626, -4.2103) (8.2684, -4.2279) (8.2744, -4.2454) (8.2805, -4.2629) (8.2867, -4.2805) (8.293, -4.298) (8.2995, -4.3155) (8.3061, -4.3331) (8.3128, -4.3506) (8.3197, -4.3681) (8.3267, -4.3856) (8.3338, -4.403) (8.341, -4.4205) (8.3484, -4.438) (8.3559, -4.4554) (8.3635, -4.4729) (8.3712, -4.4903) (8.379, -4.5077) (8.387, -4.5252) (8.395, -4.5426) (8.4032, -4.5599) (8.4115, -4.5773) (8.42, -4.5947) (8.4285, -4.612) (8.4372, -4.6293) (8.4459, -4.6467) (8.4548, -4.664) (8.4638, -4.6813) (8.4729, -4.6985) (8.4821, -4.7158) (8.4914, -4.733) (8.5009, -4.7502) (8.5104, -4.7674) (8.5201, -4.7846) (8.5298, -4.8018) (8.5397, -4.8189) (8.5497, -4.8361) (8.5598, -4.8532) (8.5679, -4.8668) (8.5741, -4.8771) (8.5782, -4.8839) (8.5803, -4.8873) knots 0 0 0 0 0 0 0.01428571 0.02857143 0.04285714 0.05714286 0.07142857 0.08571429 0.1 0.11428571 0.12857143 0.14285714 0.15714286 0.17142857 0.18571429 0.2 0.21428571 0.22857143 0.24285714 0.25714286 0.27142857 0.28571429 0.3 0.31428571 0.32857143 0.34285714 0.35714286 0.37142857 0.38571429 0.4 0.41428571 0.42857143 0.44285714 0.45714286 0.47142857 0.48571429 0.5 0.51428571 0.52857143 0.54285714 0.55714286 0.57142857 0.58571429 0.6 0.61428571 0.62857143 0.64285714 0.65714286 0.67142857 0.68571429 0.7 0.71428571 0.72857143 0.74285714 0.75714286 0.77142857 0.78571429 0.8 0.81428571 0.82857143 0.84285714 0.85714286 0.87142857 0.88571429 0.9 0.91428571 0.92857143 0.94285714 0.95714286 0.97142857 0.98571429 1 1 1 1 1 1
  arc A38 (8.5803, -4.8873) -> (9.1127, -4.8873) centre (8.8465, 2.3078) ccw
  spline S25 degree 5 poles (9.1127, -4.8873) (9.1148, -4.8839) (9.1189, -4.8771) (9.1251, -4.8668) (9.1332, -4.8532) (9.1433, -4.8361) (9.1533, -4.8189) (9.1631, -4.8018) (9.1729, -4.7846) (9.1825, -4.7674) (9.1921, -4.7502) (9.2015, -4.733) (9.2108, -4.7158) (9.2201, -4.6985) (9.2292, -4.6813) (9.2382, -4.664) (9.247, -4.6467) (9.2558, -4.6293) (9.2645, -4.612) (9.273, -4.5947) (9.2814, -4.5773) (9.2897, -4.5599) (9.2979, -4.5426) (9.306, -4.5252) (9.314, -4.5077) (9.3218, -4.4903) (9.3295, -4.4729) (9.3371, -4.4554) (9.3446, -4.438) (9.3519, -4.4205) (9.3592, -4.403) (9.3663, -4.3856) (9.3733, -4.3681) (9.3801, -4.3506) (9.3869, -4.3331) (9.3935, -4.3155) (9.3999, -4.298) (9.4063, -4.2805) (9.4125, -4.2629) (9.4186, -4.2454) (9.4245, -4.2279) (9.4303, -4.2103) (9.436, -4.1928) (9.4415, -4.1752) (9.4469, -4.1576) (9.4521, -4.1401) (9.4572, -4.1225) (9.4622, -4.1049) (9.467, -4.0874) (9.4717, -4.0698) (9.4762, -4.0522) (9.4805, -4.0347) (9.4847, -4.0171) (9.4887, -3.9995) (9.4925, -3.982) (9.4962, -3.9644) (9.4997, -3.9469) (9.5031, -3.9293) (9.5063, -3.9118) (9.5093, -3.8943) (9.5121, -3.8768) (9.5146, -3.8592) (9.5169, -3.8417) (9.5189, -3.8243) (9.5207, -3.8068) (9.5223, -3.7893) (9.5238, -3.7719) (9.5251, -3.7545) (9.5263, -3.7371) (9.5271, -3.7197) (9.5273, -3.7024) (9.5269, -3.6885) (9.5262, -3.6782) (9.5255, -3.6713) (9.5251, -3.6679) knots -1 -1 -1 -1 -1 -1 -0.98571429 -0.97142857 -0.95714286 -0.94285714 -0.92857143 -0.91428571 -0.9 -0.88571429 -0.87142857 -0.85714286 -0.84285714 -0.82857143 -0.81428571 -0.8 -0.78571429 -0.77142857 -0.75714286 -0.74285714 -0.72857143 -0.71428571 -0.7 -0.68571429 -0.67142857 -0.65714286 -0.64285714 -0.62857143 -0.61428571 -0.6 -0.58571429 -0.57142857 -0.55714286 -0.54285714 -0.52857143 -0.51428571 -0.5 -0.48571429 -0.47142857 -0.45714286 -0.44285714 -0.42857143 -0.41428571 -0.4 -0.38571429 -0.37142857 -0.35714286 -0.34285714 -0.32857143 -0.31428571 -0.3 -0.28571429 -0.27142857 -0.25714286 -0.24285714 -0.22857143 -0.21428571 -0.2 -0.18571429 -0.17142857 -0.15714286 -0.14285714 -0.12857143 -0.11428571 -0.1 -0.08571429 -0.07142857 -0.05714286 -0.04285714 -0.02857143 -0.01428571 0 0 0 0 0 0
  line L38 (9.5251, -3.6679) -> (9.4864, -3.3269)
  arc A39 (9.6555, -3.1065) -> (9.4864, -3.3269) centre (9.6851, -3.3043) ccw
  line L39 (9.6555, -3.1065) -> (10.5507, -3.1065)
  arc A40 (10.7199, -3.3269) -> (10.5507, -3.1065) centre (10.5211, -3.3043) ccw
  line L40 (10.7199, -3.3269) -> (10.6811, -3.6679)
  spline S26 degree 5 poles (10.6811, -3.6679) (10.6808, -3.6713) (10.6801, -3.6782) (10.6793, -3.6885) (10.6789, -3.7024) (10.6792, -3.7197) (10.68, -3.7371) (10.6811, -3.7545) (10.6825, -3.7719) (10.6839, -3.7893) (10.6855, -3.8068) (10.6873, -3.8243) (10.6893, -3.8417) (10.6916, -3.8592) (10.6941, -3.8768) (10.6969, -3.8943) (10.7, -3.9118) (10.7032, -3.9293) (10.7065, -3.9469) (10.71, -3.9644) (10.7137, -3.982) (10.7175, -3.9995) (10.7215, -4.0171) (10.7257, -4.0347) (10.73, -4.0522) (10.7346, -4.0698) (10.7392, -4.0874) (10.744, -4.1049) (10.749, -4.1225) (10.7541, -4.1401) (10.7593, -4.1576) (10.7647, -4.1752) (10.7702, -4.1928) (10.7759, -4.2103) (10.7817, -4.2279) (10.7877, -4.2454) (10.7937, -4.2629) (10.8, -4.2805) (10.8063, -4.298) (10.8128, -4.3155) (10.8194, -4.3331) (10.8261, -4.3506) (10.833, -4.3681) (10.84, -4.3856) (10.8471, -4.403) (10.8543, -4.4205) (10.8617, -4.438) (10.8691, -4.4554) (10.8767, -4.4729) (10.8844, -4.4903) (10.8923, -4.5077) (10.9002, -4.5252) (10.9083, -4.5426) (10.9165, -4.5599) (10.9248, -4.5773) (10.9332, -4.5947) (10.9418, -4.612) (10.9504, -4.6293) (10.9592, -4.6467) (10.9681, -4.664) (10.9771, -4.6813) (10.9862, -4.6985) (10.9954, -4.7158) (11.0047, -4.733) (11.0141, -4.7502) (11.0237, -4.7674) (11.0333, -4.7846) (11.0431, -4.8018) (11.053, -4.8189) (11.0629, -4.8361) (11.073, -4.8532) (11.0812, -4.8668) (11.0873, -4.8771) (11.0915, -4.8839) (11.0935, -4.8873) knots 0 0 0 0 0 0 0.01428571 0.02857143 0.04285714 0.05714286 0.07142857 0.08571429 0.1 0.11428571 0.12857143 0.14285714 0.15714286 0.17142857 0.18571429 0.2 0.21428571 0.22857143 0.24285714 0.25714286 0.27142857 0.28571429 0.3 0.31428571 0.32857143 0.34285714 0.35714286 0.37142857 0.38571429 0.4 0.41428571 0.42857143 0.44285714 0.45714286 0.47142857 0.48571429 0.5 0.51428571 0.52857143 0.54285714 0.55714286 0.57142857 0.58571429 0.6 0.61428571 0.62857143 0.64285714 0.65714286 0.67142857 0.68571429 0.7 0.71428571 0.72857143 0.74285714 0.75714286 0.77142857 0.78571429 0.8 0.81428571 0.82857143 0.84285714 0.85714286 0.87142857 0.88571429 0.9 0.91428571 0.92857143 0.94285714 0.95714286 0.97142857 0.98571429 1 1 1 1 1 1
  arc A41 (11.0935, -4.8873) -> (11.626, -4.8873) centre (11.3598, 2.3078) ccw
  spline S27 degree 5 poles (11.626, -4.8873) (11.628, -4.8839) (11.6322, -4.8771) (11.6383, -4.8668) (11.6465, -4.8532) (11.6566, -4.8361) (11.6665, -4.8189) (11.6764, -4.8018) (11.6862, -4.7846) (11.6958, -4.7674) (11.7054, -4.7502) (11.7148, -4.733) (11.7241, -4.7158) (11.7333, -4.6985) (11.7424, -4.6813) (11.7514, -4.664) (11.7603, -4.6467) (11.7691, -4.6293) (11.7777, -4.612) (11.7863, -4.5947) (11.7947, -4.5773) (11.803, -4.5599) (11.8112, -4.5426) (11.8193, -4.5252) (11.8272, -4.5077) (11.8351, -4.4903) (11.8428, -4.4729) (11.8504, -4.4554) (11.8579, -4.438) (11.8652, -4.4205) (11.8725, -4.403) (11.8796, -4.3856) (11.8865, -4.3681) (11.8934, -4.3506) (11.9001, -4.3331) (11.9067, -4.3155) (11.9132, -4.298) (11.9196, -4.2805) (11.9258, -4.2629) (11.9318, -4.2454) (11.9378, -4.2279) (11.9436, -4.2103) (11.9493, -4.1928) (11.9548, -4.1752) (11.9602, -4.1576) (11.9654, -4.1401) (11.9705, -4.1225) (11.9755, -4.1049) (11.9803, -4.0874) (11.985, -4.0698) (11.9895, -4.0522) (11.9938, -4.0347) (11.998, -4.0171) (12.002, -3.9995) (12.0058, -3.982) (12.0095, -3.9644) (12.013, -3.9469) (12.0164, -3.9293) (12.0196, -3.9118) (12.0226, -3.8943) (12.0254, -3.8768) (12.0279, -3.8592) (12.0302, -3.8417) (12.0322, -3.8243) (12.034, -3.8068) (12.0356, -3.7893) (12.037, -3.7719) (12.0384, -3.7545) (12.0395, -3.7371) (12.0403, -3.7197) (12.0406, -3.7024) (12.0402, -3.6885) (12.0394, -3.6782) (12.0388, -3.6713) (12.0384, -3.6679) knots -1 -1 -1 -1 -1 -1 -0.98571429 -0.97142857 -0.95714286 -0.94285714 -0.92857143 -0.91428571 -0.9 -0.88571429 -0.87142857 -0.85714286 -0.84285714 -0.82857143 -0.81428571 -0.8 -0.78571429 -0.77142857 -0.75714286 -0.74285714 -0.72857143 -0.71428571 -0.7 -0.68571429 -0.67142857 -0.65714286 -0.64285714 -0.62857143 -0.61428571 -0.6 -0.58571429 -0.57142857 -0.55714286 -0.54285714 -0.52857143 -0.51428571 -0.5 -0.48571429 -0.47142857 -0.45714286 -0.44285714 -0.42857143 -0.41428571 -0.4 -0.38571429 -0.37142857 -0.35714286 -0.34285714 -0.32857143 -0.31428571 -0.3 -0.28571429 -0.27142857 -0.25714286 -0.24285714 -0.22857143 -0.21428571 -0.2 -0.18571429 -0.17142857 -0.15714286 -0.14285714 -0.12857143 -0.11428571 -0.1 -0.08571429 -0.07142857 -0.05714286 -0.04285714 -0.02857143 -0.01428571 0 0 0 0 0 0
  line L41 (12.0384, -3.6679) -> (11.9996, -3.3269)
  arc A42 (12.1688, -3.1065) -> (11.9996, -3.3269) centre (12.1984, -3.3043) ccw
  line L42 (12.1688, -3.1065) -> (13.064, -3.1065)
  arc A43 (13.2331, -3.3269) -> (13.064, -3.1065) centre (13.0344, -3.3043) ccw
  line L43 (13.2331, -3.3269) -> (13.1944, -3.6679)
  spline S28 degree 5 poles (13.1944, -3.6679) (13.194, -3.6713) (13.1933, -3.6782) (13.1926, -3.6885) (13.1922, -3.7024) (13.1924, -3.7197) (13.1932, -3.7371) (13.1944, -3.7545) (13.1957, -3.7719) (13.1972, -3.7893) (13.1988, -3.8068) (13.2006, -3.8243) (13.2026, -3.8417) (13.2049, -3.8592) (13.2074, -3.8768) (13.2102, -3.8943) (13.2132, -3.9118) (13.2164, -3.9293) (13.2198, -3.9469) (13.2233, -3.9644) (13.227, -3.982) (13.2308, -3.9995) (13.2348, -4.0171) (13.239, -4.0347) (13.2433, -4.0522) (13.2478, -4.0698) (13.2525, -4.0874) (13.2573, -4.1049) (13.2623, -4.1225) (13.2674, -4.1401) (13.2726, -4.1576) (13.278, -4.1752) (13.2835, -4.1928) (13.2892, -4.2103) (13.295, -4.2279) (13.3009, -4.2454) (13.307, -4.2629) (13.3132, -4.2805) (13.3196, -4.298) (13.3261, -4.3155) (13.3327, -4.3331) (13.3394, -4.3506) (13.3462, -4.3681) (13.3532, -4.3856) (13.3603, -4.403) (13.3676, -4.4205) (13.3749, -4.438) (13.3824, -4.4554) (13.39, -4.4729) (13.3977, -4.4903) (13.4056, -4.5077) (13.4135, -4.5252) (13.4216, -4.5426) (13.4298, -4.5599) (13.4381, -4.5773) (13.4465, -4.5947) (13.4551, -4.612) (13.4637, -4.6293) (13.4725, -4.6467) (13.4814, -4.664) (13.4903, -4.6813) (13.4995, -4.6985) (13.5087, -4.7158) (13.518, -4.733) (13.5274, -4.7502) (13.537, -4.7674) (13.5466, -4.7846) (13.5564, -4.8018) (13.5662, -4.8189) (13.5762, -4.8361) (13.5863, -4.8532) (13.5945, -4.8668) (13.6006, -4.8771) (13.6047, -4.8839) (13.6068, -4.8873) knots 0 0 0 0 0 0 0.01428571 0.02857143 0.04285714 0.05714286 0.07142857 0.08571429 0.1 0.11428571 0.12857143 0.14285714 0.15714286 0.17142857 0.18571429 0.2 0.21428571 0.22857143 0.24285714 0.25714286 0.27142857 0.28571429 0.3 0.31428571 0.32857143 0.34285714 0.35714286 0.37142857 0.38571429 0.4 0.41428571 0.42857143 0.44285714 0.45714286 0.47142857 0.48571429 0.5 0.51428571 0.52857143 0.54285714 0.55714286 0.57142857 0.58571429 0.6 0.61428571 0.62857143 0.64285714 0.65714286 0.67142857 0.68571429 0.7 0.71428571 0.72857143 0.74285714 0.75714286 0.77142857 0.78571429 0.8 0.81428571 0.82857143 0.84285714 0.85714286 0.87142857 0.88571429 0.9 0.91428571 0.92857143 0.94285714 0.95714286 0.97142857 0.98571429 1 1 1 1 1 1
  arc A44 (13.6068, -4.8873) -> (14.1393, -4.8873) centre (13.873, 2.3078) ccw
  spline S29 degree 5 poles (14.1393, -4.8873) (14.1413, -4.8839) (14.1454, -4.8771) (14.1516, -4.8668) (14.1598, -4.8532) (14.1698, -4.8361) (14.1798, -4.8189) (14.1897, -4.8018) (14.1994, -4.7846) (14.2091, -4.7674) (14.2186, -4.7502) (14.2281, -4.733) (14.2374, -4.7158) (14.2466, -4.6985) (14.2557, -4.6813) (14.2647, -4.664) (14.2736, -4.6467) (14.2824, -4.6293) (14.291, -4.612) (14.2995, -4.5947) (14.308, -4.5773) (14.3163, -4.5599) (14.3245, -4.5426) (14.3325, -4.5252) (14.3405, -4.5077) (14.3483, -4.4903) (14.3561, -4.4729) (14.3637, -4.4554) (14.3711, -4.438) (14.3785, -4.4205) (14.3857, -4.403) (14.3928, -4.3856) (14.3998, -4.3681) (14.4067, -4.3506) (14.4134, -4.3331) (14.42, -4.3155) (14.4265, -4.298) (14.4328, -4.2805) (14.439, -4.2629) (14.4451, -4.2454) (14.4511, -4.2279) (14.4569, -4.2103) (14.4625, -4.1928) (14.4681, -4.1752) (14.4734, -4.1576) (14.4787, -4.1401) (14.4838, -4.1225) (14.4888, -4.1049) (14.4936, -4.0874) (14.4982, -4.0698) (14.5027, -4.0522) (14.5071, -4.0347) (14.5112, -4.0171) (14.5152, -3.9995) (14.5191, -3.982) (14.5227, -3.9644) (14.5263, -3.9469) (14.5296, -3.9293) (14.5328, -3.9118) (14.5359, -3.8943) (14.5387, -3.8768) (14.5412, -3.8592) (14.5435, -3.8417) (14.5455, -3.8243) (14.5472, -3.8068) (14.5488, -3.7893) (14.5503, -3.7719) (14.5517, -3.7545) (14.5528, -3.7371) (14.5536, -3.7197) (14.5539, -3.7024) (14.5534, -3.6885) (14.5527, -3.6782) (14.552, -3.6713) (14.5516, -3.6679) knots -1 -1 -1 -1 -1 -1 -0.98571429 -0.97142857 -0.95714286 -0.94285714 -0.92857143 -0.91428571 -0.9 -0.88571429 -0.87142857 -0.85714286 -0.84285714 -0.82857143 -0.81428571 -0.8 -0.78571429 -0.77142857 -0.75714286 -0.74285714 -0.72857143 -0.71428571 -0.7 -0.68571429 -0.67142857 -0.65714286 -0.64285714 -0.62857143 -0.61428571 -0.6 -0.58571429 -0.57142857 -0.55714286 -0.54285714 -0.52857143 -0.51428571 -0.5 -0.48571429 -0.47142857 -0.45714286 -0.44285714 -0.42857143 -0.41428571 -0.4 -0.38571429 -0.37142857 -0.35714286 -0.34285714 -0.32857143 -0.31428571 -0.3 -0.28571429 -0.27142857 -0.25714286 -0.24285714 -0.22857143 -0.21428571 -0.2 -0.18571429 -0.17142857 -0.15714286 -0.14285714 -0.12857143 -0.11428571 -0.1 -0.08571429 -0.07142857 -0.05714286 -0.04285714 -0.02857143 -0.01428571 0 0 0 0 0 0
  line L44 (14.5516, -3.6679) -> (14.5129, -3.3269)
  arc A45 (14.6821, -3.1065) -> (14.5129, -3.3269) centre (14.7116, -3.3043) ccw
  line L45 (14.6821, -3.1065) -> (15.5772, -3.1065)
  arc A46 (15.7464, -3.3269) -> (15.5772, -3.1065) centre (15.5477, -3.3043) ccw
  line L46 (15.7464, -3.3269) -> (15.7077, -3.6679)
  spline S30 degree 5 poles (15.7077, -3.6679) (15.7073, -3.6713) (15.7066, -3.6782) (15.7059, -3.6885) (15.7055, -3.7024) (15.7057, -3.7197) (15.7065, -3.7371) (15.7077, -3.7545) (15.709, -3.7719) (15.7105, -3.7893) (15.7121, -3.8068) (15.7139, -3.8243) (15.7159, -3.8417) (15.7181, -3.8592) (15.7207, -3.8768) (15.7235, -3.8943) (15.7265, -3.9118) (15.7297, -3.9293) (15.7331, -3.9469) (15.7366, -3.9644) (15.7403, -3.982) (15.7441, -3.9995) (15.7481, -4.0171) (15.7523, -4.0347) (15.7566, -4.0522) (15.7611, -4.0698) (15.7658, -4.0874) (15.7706, -4.1049) (15.7755, -4.1225) (15.7806, -4.1401) (15.7859, -4.1576) (15.7913, -4.1752) (15.7968, -4.1928) (15.8025, -4.2103) (15.8083, -4.2279) (15.8142, -4.2454) (15.8203, -4.2629) (15.8265, -4.2805) (15.8329, -4.298) (15.8393, -4.3155) (15.8459, -4.3331) (15.8527, -4.3506) (15.8595, -4.3681) (15.8665, -4.3856) (15.8736, -4.403) (15.8808, -4.4205) (15.8882, -4.438) (15.8957, -4.4554) (15.9033, -4.4729) (15.911, -4.4903) (15.9188, -4.5077) (15.9268, -4.5252) (15.9349, -4.5426) (15.9431, -4.5599) (15.9514, -4.5773) (15.9598, -4.5947) (15.9683, -4.612) (15.977, -4.6293) (15.9858, -4.6467) (15.9946, -4.664) (16.0036, -4.6813) (16.0127, -4.6985) (16.0219, -4.7158) (16.0313, -4.733) (16.0407, -4.7502) (16.0502, -4.7674) (16.0599, -4.7846) (16.0697, -4.8018) (16.0795, -4.8189) (16.0895, -4.8361) (16.0996, -4.8532) (16.1077, -4.8668) (16.1139, -4.8771) (16.118, -4.8839) (16.1201, -4.8873) knots 0 0 0 0 0 0 0.01428571 0.02857143 0.04285714 0.05714286 0.07142857 0.08571429 0.1 0.11428571 0.12857143 0.14285714 0.15714286 0.17142857 0.18571429 0.2 0.21428571 0.22857143 0.24285714 0.25714286 0.27142857 0.28571429 0.3 0.31428571 0.32857143 0.34285714 0.35714286 0.37142857 0.38571429 0.4 0.41428571 0.42857143 0.44285714 0.45714286 0.47142857 0.48571429 0.5 0.51428571 0.52857143 0.54285714 0.55714286 0.57142857 0.58571429 0.6 0.61428571 0.62857143 0.64285714 0.65714286 0.67142857 0.68571429 0.7 0.71428571 0.72857143 0.74285714 0.75714286 0.77142857 0.78571429 0.8 0.81428571 0.82857143 0.84285714 0.85714286 0.87142857 0.88571429 0.9 0.91428571 0.92857143 0.94285714 0.95714286 0.97142857 0.98571429 1 1 1 1 1 1
  arc A47 (16.1201, -4.8873) -> (16.6525, -4.8873) centre (16.3863, 2.3078) ccw
  spline S31 degree 5 poles (16.6525, -4.8873) (16.6546, -4.8839) (16.6587, -4.8771) (16.6649, -4.8668) (16.673, -4.8532) (16.6831, -4.8361) (16.6931, -4.8189) (16.703, -4.8018) (16.7127, -4.7846) (16.7224, -4.7674) (16.7319, -4.7502) (16.7413, -4.733) (16.7507, -4.7158) (16.7599, -4.6985) (16.769, -4.6813) (16.778, -4.664) (16.7869, -4.6467) (16.7956, -4.6293) (16.8043, -4.612) (16.8128, -4.5947) (16.8212, -4.5773) (16.8295, -4.5599) (16.8377, -4.5426) (16.8458, -4.5252) (16.8538, -4.5077) (16.8616, -4.4903) (16.8693, -4.4729) (16.8769, -4.4554) (16.8844, -4.438) (16.8918, -4.4205) (16.899, -4.403) (16.9061, -4.3856) (16.9131, -4.3681) (16.92, -4.3506) (16.9267, -4.3331) (16.9333, -4.3155) (16.9398, -4.298) (16.9461, -4.2805) (16.9523, -4.2629) (16.9584, -4.2454) (16.9643, -4.2279) (16.9701, -4.2103) (16.9758, -4.1928) (16.9813, -4.1752) (16.9867, -4.1576) (16.992, -4.1401) (16.9971, -4.1225) (17.002, -4.1049) (17.0068, -4.0874) (17.0115, -4.0698) (17.016, -4.0522) (17.0204, -4.0347) (17.0245, -4.0171) (17.0285, -3.9995) (17.0323, -3.982) (17.036, -3.9644) (17.0395, -3.9469) (17.0429, -3.9293) (17.0461, -3.9118) (17.0491, -3.8943) (17.0519, -3.8768) (17.0545, -3.8592) (17.0567, -3.8417) (17.0587, -3.8243) (17.0605, -3.8068) (17.0621, -3.7893) (17.0636, -3.7719) (17.0649, -3.7545) (17.0661, -3.7371) (17.0669, -3.7197) (17.0671, -3.7024) (17.0667, -3.6885) (17.066, -3.6782) (17.0653, -3.6713) (17.0649, -3.6679) knots -1 -1 -1 -1 -1 -1 -0.98571429 -0.97142857 -0.95714286 -0.94285714 -0.92857143 -0.91428571 -0.9 -0.88571429 -0.87142857 -0.85714286 -0.84285714 -0.82857143 -0.81428571 -0.8 -0.78571429 -0.77142857 -0.75714286 -0.74285714 -0.72857143 -0.71428571 -0.7 -0.68571429 -0.67142857 -0.65714286 -0.64285714 -0.62857143 -0.61428571 -0.6 -0.58571429 -0.57142857 -0.55714286 -0.54285714 -0.52857143 -0.51428571 -0.5 -0.48571429 -0.47142857 -0.45714286 -0.44285714 -0.42857143 -0.41428571 -0.4 -0.38571429 -0.37142857 -0.35714286 -0.34285714 -0.32857143 -0.31428571 -0.3 -0.28571429 -0.27142857 -0.25714286 -0.24285714 -0.22857143 -0.21428571 -0.2 -0.18571429 -0.17142857 -0.15714286 -0.14285714 -0.12857143 -0.11428571 -0.1 -0.08571429 -0.07142857 -0.05714286 -0.04285714 -0.02857143 -0.01428571 0 0 0 0 0 0
  line L47 (17.0649, -3.6679) -> (17.0262, -3.3269)
  arc A48 (17.1954, -3.1065) -> (17.0262, -3.3269) centre (17.2249, -3.3043) ccw
  line L48 (17.1954, -3.1065) -> (18.0905, -3.1065)
  arc A49 (18.2597, -3.3269) -> (18.0905, -3.1065) centre (18.061, -3.3043) ccw
  line L49 (18.2597, -3.3269) -> (18.221, -3.6679)